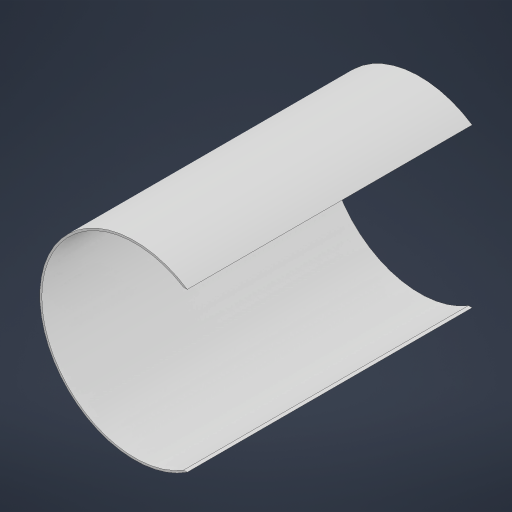
# Autodesk Inventor part: sf_Cylinder_Lagging_1
Saved by Autodesk Inventor 2024 (Build 280153000, 153)
## iProperties
Created: 2024-03-22
Part Number: sf_Cylinder_Lagging_1
Material: Generisch
Document SubType Name: Modeling
Designer: Simon
Density: 1 g/cm^3
Appearance: Vorgabe
Author: Simon
Autodesk Inventor part; units mm, degrees
ref_plane "YZ Plane" through (0, 0, 0) normal (1, 0, 0) x (0, 1, 0)
ref_plane "XZ Plane" through (0, 0, 0) normal (0, 1, 0) x (-1, 0, 0)
ref_plane "XY Plane" through (0, 0, 0) normal (0, 0, 1) x (1, 0, 0)
sketch "Skizze1" plane through (0, 0, 0) normal (0, 1, 0) x (-1, 0, 0)
  circle A0 centre (0, 0) radius 23.5
  line L0 (-34.661, -20) -> (-12.339, -20)
  line L1 (-12.339, -20) -> (-12.339, 20)
  line L2 (-12.339, 20) -> (-34.661, 20)
  line L3 (-34.661, 20) -> (-34.661, -20)
  circle A1 centre (0, 0) radius 24
  point P0 (-23.5, 0)
  point P1 (-13.2665, 20)
  point P2 (-13.2665, -20)
  dimension "d0" = 47
  dimension "d1" = 40
  dimension "d2" = 0.5
  constraints: 8 end point, 2 centre point, 2 parallel, 2 point on circle, 1 coincident, 1 horizontal, 1 perpendicular
  measures "d0" diameter of A0
  measures "d1" distance of L1.end L0.end
  measures "d2" radial gap between concentric circles of A0 A1
extrude "Extrusion1" add sketch "Skizze1" along normal blind 72 contours A0 L2 A1 L0 picked at (-9.2672, 21.6358)
